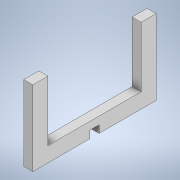
# Autodesk Inventor part: CONTAINERHOUDER KORT
Saved by Autodesk Inventor 2021 (Build 250183000, 183)
## iProperties
Created: 2022-02-02
Part Number: CONTAINERHOUDER KORT
Material: Generic
Document SubType Name: Modeling
Designer: ryan
Density: 1 g/cm^3
Appearance: Default
Author: ryan
Autodesk Inventor part; units mm, degrees
ref_plane "YZ Plane" through (0, 0, 0) normal (1, 0, 0) x (0, 1, 0)
ref_plane "XZ Plane" through (0, 0, 0) normal (0, 1, 0) x (-1, 0, 0)
ref_plane "XY Plane" through (0, 0, 0) normal (0, 0, 1) x (1, 0, 0)
sketch "Sketch1" plane through (0, 0, 0) normal (1, 0, 0) x (0, 1, 0)
  line L0 (0, 0) -> (0, 31)
  line L1 (0, 31) -> (20, 31)
  line L2 (20, 31) -> (20, 36)
  line L3 (20, 36) -> (-5, 36)
  line L4 (-5, 36) -> (-5, 0)
  line L5 (-5, 0) -> (20, 0)
  line L6 (20, 0) -> (20, -5)
  line L7 (20, -5) -> (-5, -5)
  line L8 (-5, -5) -> (-5, 0)
  line L9 (0, 15.5) -> (0, 17)
  line L10 (0, 17) -> (-2.5, 17)
  line L11 (-2.5, 17) -> (-2.5, 14)
  line L12 (-2.5, 14) -> (0, 14)
  line L13 (0, 14) -> (0, 17)
  line L14 (-2.5, 17) -> (-5, 17)
  line L15 (-2.5, 17) -> (-5, 17)
  line L16 (-5, 17) -> (-5, 14)
  line L17 (-5, 14) -> (-2.5, 14)
  line L18 (-2.5, 14) -> (-2.5, 17)
  dimension "d0" = 31
  dimension "d1" = 20
  dimension "d2" = 5
  dimension "d3" = 25
  dimension "d5" = 25
  dimension "d6" = 5
  dimension "d7" = 1.5
  dimension "d8" = 2.5
  dimension "d9" = 3
  constraints: 38 end point, 7 perpendicular, 6 parallel, 4 horizontal, 3 point on line, 1 midpoint, 1 vertical
  measures "d0" distance of L0.start L0.end
  measures "d1" distance of L0.end L1.end
  measures "d2" distance of L1.end L2.end
  measures "d3" distance of L2.end L3.end
  measures "d5" distance of L6.end L7.end
  measures "d6" distance of L5.end L6.end
  measures "d7" distance of L9.start L9.end
  measures "d8" distance of L12.end L11.end
  measures "d9" distance of L11.end L10.end
extrude "Extrusion1" add sketch "Sketch1" along normal blind 3 contours L5 L4 L17 L12 L0 | L5 L6 L7 L8 | L12 L11 L10 L0 | L10 L14 L4 L3 L2 L1 L0
body "Solid1"
